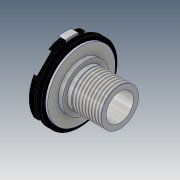
# Autodesk Inventor part: Plug P10 femea
Saved by Autodesk Inventor 2016 (Build 200138000, 138)
## iProperties
Created: 2018-12-01
Part Number: Plug P10 femea
Material: Generic
Document SubType Name: Modeling
Designer: Pedro Mendonça
Density: 1 g/cm^3
Appearance: Aluminum - Flat
Author: Pedro Mendonça
Autodesk Inventor part; units mm, degrees
ref_plane "YZ Plane" through (0, 0, 0) normal (1, 0, 0) x (0, 1, 0)
ref_plane "XZ Plane" through (0, 0, 0) normal (0, 1, 0) x (-1, 0, 0)
ref_plane "XY Plane" through (0, 0, 0) normal (0, 0, 1) x (1, 0, 0)
sketch "Sketch1" plane through (0, 0, 0) normal (0, 1, 0) x (-1, 0, 0)
  circle A0 centre (0, 0) radius 4.4
  dimension "d0" = 8.8
  constraints: 1 centre point, 1 coincident
  measures "d0" diameter of A0
extrude "Extrusion1" add sketch "Sketch1" against normal blind 7
sketch "Sketch2" plane through (0, 0, 0) normal (0, 1, 0) x (1, 0, 0)
  circle A0 centre (0, 0) radius 3.3
  dimension "d3" = 6.6
  constraints: 1 centre point, 1 coincident
  measures "d3" diameter of A0
thread "Thread1" size "M9x0.75" class "6g" standard "ANSI Metric M Profile" full length
sketch "Sketch3" plane through (0, -7, 0) normal (0, -1, 0) x (1, 0, 0)
  circle A0 centre (0, 0) radius 4.4 projected
extrude "Extrusion2" add sketch "Sketch3" along normal blind 1 separate body
sketch "Sketch4" plane through (0, -8, 0) normal (0, -1, 0) x (1, 0, 0)
  circle A0 centre (0, 0) radius 5.45
  dimension "d8" = 10.9
  constraints: 1 centre point, 1 coincident
  measures "d8" diameter of A0
extrude "Extrusion3" add sketch "Sketch4" along normal blind 1 bodies 2
sketch "Sketch5" plane through (0, -9, 0) normal (0, -1, 0) x (1, 0, 0)
  circle A0 centre (0, 0) radius 7.95
  dimension "d11" = 15.9
  constraints: 1 centre point, 1 coincident
  measures "d11" diameter of A0
extrude "Extrusion4" add sketch "Sketch5" along normal blind 0.5 bodies 2
sketch "Sketch6" plane through (0, -9.5, 0) normal (0, -1, 0) x (1, 0, 0)
  circle A0 centre (0, 0) radius 8.9
  dimension "d14" = 17.8
  constraints: 1 centre point, 1 coincident
  measures "d14" diameter of A0
extrude "Extrusion5" add sketch "Sketch6" along normal blind 1.2 separate body
sketch "Sketch7" plane through (0, -10.7, 0) normal (0, -1, 0) x (1, 0, 0)
  circle A0 centre (0, 0) radius 7.5
  dimension "d17" = 15
  constraints: 1 centre point, 1 coincident
  measures "d17" diameter of A0
extrude "Extrusion6" add sketch "Sketch7" along normal blind 0.5 separate body
sketch "Sketch8" plane through (0, -11.2, 0) normal (0, -1, 0) x (1, 0, 0)
  circle A0 centre (0, 0) radius 8.9 projected
extrude "Extrusion7" add sketch "Sketch8" along normal blind 1.2 separate body
sketch "Sketch9" plane through (0, -12.4, 0) normal (0, -1, 0) x (1, 0, 0)
  circle A0 centre (0, 0) radius 8.9 projected
extrude "Extrusion8" add sketch "Sketch9" along normal blind 0.5 bodies 1
sketch "Sketch10" plane through (0, -12.9, 0) normal (0, -1, 0) x (1, 0, 0)
  line L0 (-5.1426, -7.2639) -> (-4.4355, -6.5568)
  line L1 (-4.4355, -6.5568) -> (-6.5568, -4.4355)
  line L2 (-4.4355, -6.5568) -> (-5.1426, -7.2639)
  line L3 (-6.5568, -4.4355) -> (-7.2639, -5.1426)
  line L4 (4.4978, -7.6798) -> (3.7907, -6.9727)
  line L5 (3.7907, -6.9727) -> (6.9727, -3.7907)
  line L6 (6.9727, -3.7907) -> (7.6798, -4.4978)
  line L7 (3.7907, -6.9727) -> (4.4978, -7.6798)
  line L8 (7.7572, 4.3631) -> (7.0501, 3.656)
  line L9 (7.0501, 3.656) -> (3.6361, 7.0699)
  line L10 (7.0501, 3.656) -> (7.7572, 4.3631)
  line L11 (3.6361, 7.0699) -> (4.3631, 7.7572)
  line L12 (-3.0557, 8.359) -> (-2.3486, 7.6519)
  line L13 (-2.3486, 7.6519) -> (-7.6519, 2.3486)
  line L14 (-2.3486, 7.6519) -> (-3.0557, 8.359)
  line L15 (-7.6519, 2.3486) -> (-8.359, 3.0557)
  arc A0 (-7.2639, -5.1426) -> (-5.1426, -7.2639) centre (0, 0) ccw
  arc A1 (4.4978, -7.6798) -> (7.6798, -4.4978) centre (0, 0) ccw
  arc A2 (7.7572, 4.3631) -> (4.3631, 7.7572) centre (0, 0) ccw
  arc A3 (-3.0557, 8.359) -> (-8.359, 3.0557) centre (0, 0) ccw
  line L16 (1.5, 7.7727) -> (1.5, 8.7727)
  line L17 (-1.5, 7.7727) -> (-1.5, 8.7727)
  line L18 (2.25, -7.6109) -> (2.25, -8.6109)
  line L19 (-2.25, -7.6109) -> (-2.25, -8.6109)
  arc A4 (-2.25, -8.6109) -> (2.25, -8.6109) centre (0, 0) ccw
  arc A5 (-7.2639, -5.1426) -> (-5.1426, -7.2639) centre (0, 0) ccw
  arc A6 (4.4978, -7.6798) -> (7.6798, -4.4978) centre (0, 0) ccw
  arc A7 (7.7572, 4.3631) -> (4.3631, 7.7572) centre (0, 0) ccw
  arc A8 (1.5, 8.7727) -> (-1.5, 8.7727) centre (0, 0) ccw
  arc A9 (-3.0557, 8.359) -> (-8.359, 3.0557) centre (0, 0) ccw
  line L20 (-1.5, 8.7727) -> (-1.5, 7.7727)
  line L21 (-1.5, 7.7727) -> (1.5, 7.7727)
  line L22 (2.25, -8.6109) -> (2.25, -7.6109)
  line L23 (2.25, -7.6109) -> (-2.25, -7.6109)
  dimension "d38" = 1
  dimension "d39" = 1
  dimension "d40" = 1
  dimension "d42" = 1
  dimension "d49" = 1
  dimension "d50" = 1
  constraints: 48 end point, 23 point on circle, 10 centre point, 5 perpendicular, 5 other
  measures "d38" distance of L0.start L0.end
  measures "d39" distance of L4.start L4.end
  measures "d40" distance of L8.start L8.end
  measures "d42" distance of L12.start L12.end
  measures "d49" distance of L17.start L17.end
  measures "d50" distance of L18.start L18.end
extrude "Extrusion9" cut sketch "Sketch10" against normal blind 1.7 bodies 5
extrude "Extrusion10" cut sketch "Sketch2" against normal through all bodies 1 2 3 4 5 6
sketch "Sketch11" plane through (0, 0, 0) normal (0, 1, 0) x (1, 0, 0)
  circle A0 centre (0, 0) radius 3.3 projected
  circle A1 centre (0, 0) radius 3.2
  dimension "d53" = 0.1
  constraints: 1 centre point
  measures "d53" radial gap between concentric circles of A0 A1
extrude "Extrusion11" add sketch "Sketch11" against normal blind 14 bodies 1
fillet "Fillet1" radius 0.5 1 edges at (-3.3, -12.9, 0)
sketch "Sketch12" plane through (0, -12.9, 0) normal (0, -1, 0) x (1, 0, 0)
  arc A0 (-5.9, 0) -> (5.9, 0) centre (0, 0) ccw
  circle A1 centre (0, 0) radius 8.9
  line L0 (-1.5, 8.7727) -> (-1.5, 7.7727)
  line L1 (-1.5, 7.7727) -> (1.5, 7.7727) construction
  line L2 (-1.5, 7.7727) -> (-1.5, 8.7727)
  line L3 (1.5, 7.7727) -> (1.5, 8.7727)
  line L4 (-1.5, 7.7727) -> (-5.9, 0)
  line L5 (0, 0) -> (0, 1.7918) construction
  line L6 (1.5, 7.7727) -> (5.9, 0)
  dimension "d57" = 11.8
  dimension "d60" = 1
  constraints: 14 end point, 4 point on circle, 2 centre point, 1 coincident, 1 perpendicular, 1 symmetric about line, 1 vertical
  measures "d57" diameter of A0
  measures "d60" distance of L0.start L0.end
extrude "Extrusion12" cut sketch "Sketch12" against normal blind 0.5 contours A0 L6 L3 A1 L0 L4 picked at (-4.2563, 4.957) bodies 1
sketch "Sketch13" plane through (0, -12.4, 0) normal (0, 1, 0) x (1, 0, 0)
  circle A0 centre (0, 0) radius 8.9 projected
  line L0 (1.5, -7.7727) -> (1.5, -8.7727) projected
  line L1 (-1.5, -8.7727) -> (-1.5, -7.7727) projected
  line L2 (-1.5, -7.7727) -> (1.5, -7.7727) projected
extrude "Extrusion13" add sketch "Sketch13" along normal blind 1.2 contours L1 L2 L0 A0 picked at (0.1674, -8.1437) bodies 1
ref_plane "Work Plane1" through (3.0836, -12.4, -6.2656) normal (0.7071068, 0, -0.7071068) x (-0.7071068, 0, -0.7071068)
sketch "Sketch14" plane through (3.0836, -12.4, -6.2656) normal (0.7071068, 0, -0.7071068) x (-0.7071068, 0, -0.7071068)
  line L0 (-4.5, 0) -> (-4.5, 1.2) projected
  line L1 (-4.5, 1.2) -> (-4.5, 1.7)
  line L2 (-11.15, 1.7) -> (6.65, 1.7) projected
  line L3 (0, 0) -> (0, 1.2) projected
  line L4 (0, 1.2) -> (0, 1.7)
  line L5 (-4.5, 1.7) -> (0, 1.7)
  line L6 (-4.5, 1.2) -> (0, 1.2)
  line L7 (1.5, 1.2) -> (-6, 1.2) projected
  point P0 (-2.25, 12.4)
  constraints: 8 end point, 3 collinear, 2 point on line, 1 perpendicular
extrude "Extrusion14" add sketch "Sketch14" along normal blind 1.8 bodies 4
ref_plane "Work Plane2" through (-3.0557, -12.4, 8.359) normal (-0.7071068, 0, 0.7071068) x (0.7071068, 0, 0.7071068)
sketch "Sketch15" plane through (-3.0557, -12.4, 8.359) normal (-0.7071068, 0, 0.7071068) x (0.7071068, 0, 0.7071068)
  line L0 (0, 0) -> (0, 1.2) projected
  line L1 (0, 1.2) -> (0, 1.7)
  line L2 (-12.65, 1.7) -> (5.15, 1.7) projected
  line L3 (-7.5, 0) -> (-7.5, 1.2) projected
  line L4 (-7.5, 1.2) -> (-7.5, 1.7)
  line L5 (-7.5, 1.2) -> (0, 1.2)
  line L6 (-6, 1.2) -> (-8.2478, 1.2) projected
  line L7 (-7.5, 1.7) -> (0, 1.7)
  point P0 (-3.75, 12.4)
  constraints: 8 end point, 3 point on line, 2 collinear
extrude "Extrusion15" add sketch "Sketch15" against normal up to next bodies 4
body "Solid1"
body "Solid2"
body "Solid3"
body "Solid4"
body "Solid5"
body "Solid6"
